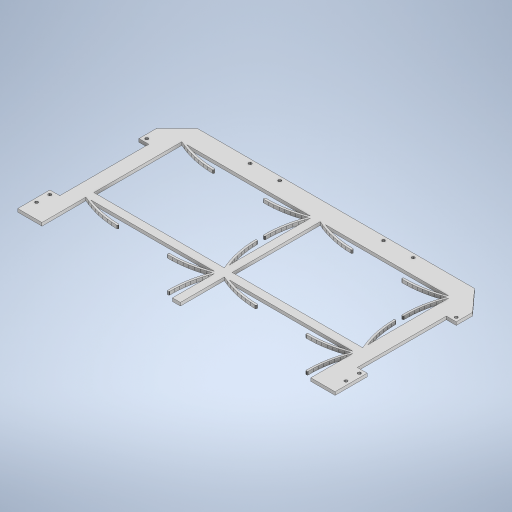
# Autodesk Inventor part: deck_bottom
Saved by Autodesk Inventor 2024.1 (Build 281209000, 209)
## iProperties
Created: 2024-06-24
Part Number: deck_bottom
Material: Generic
Document SubType Name: Modeling
Designer: pab2
Density: 1 g/cm^3
Appearance: Default
Author: pab2
Autodesk Inventor part; units mm, degrees
ref_plane "YZ Plane" through (0, 0, 0) normal (1, 0, 0) x (0, 1, 0)
ref_plane "XZ Plane" through (0, 0, 0) normal (0, 1, 0) x (-1, 0, 0)
ref_plane "XY Plane" through (0, 0, 0) normal (0, 0, 1) x (1, 0, 0)
sketch "Sketch1" plane through (0, 0, 0) normal (0, 1, 0) x (-1, 0, 0)
  line L0 (350.8022, 552.9792) -> (351.4019, 553.085)
  line L1 (351.4019, 553.085) -> (351.8958, 553.4378)
  line L2 (351.8958, 553.4378) -> (352.2133, 553.8964)
  line L3 (352.2133, 553.8964) -> (352.3192, 554.4961)
  line L4 (352.3192, 554.4961) -> (352.2133, 555.0605)
  line L5 (352.2133, 555.0605) -> (351.8958, 555.5544)
  line L6 (351.8958, 555.5544) -> (351.4019, 555.8719)
  line L7 (351.4019, 555.8719) -> (350.8022, 555.9778)
  line L8 (350.8022, 555.9778) -> (350.2378, 555.8719)
  line L9 (350.2378, 555.8719) -> (349.7439, 555.5544)
  line L10 (349.7439, 555.5544) -> (349.4264, 555.0605)
  line L11 (349.4264, 555.0605) -> (349.3206, 554.4961)
  line L12 (349.3206, 554.4961) -> (349.4264, 553.8964)
  line L13 (349.4264, 553.8964) -> (349.7439, 553.4378)
  line L14 (349.7439, 553.4378) -> (350.2378, 553.085)
  line L15 (350.2378, 553.085) -> (350.8022, 552.9792)
  line L16 (320.8161, 552.9792) -> (321.3806, 553.085)
  line L17 (321.3806, 553.085) -> (321.8745, 553.4378)
  line L18 (321.8745, 553.4378) -> (322.1919, 553.8964)
  line L19 (322.1919, 553.8964) -> (322.3331, 554.4961)
  line L20 (322.3331, 554.4961) -> (322.1919, 555.0605)
  line L21 (322.1919, 555.0605) -> (321.8745, 555.5544)
  line L22 (321.8745, 555.5544) -> (321.3806, 555.8719)
  line L23 (321.3806, 555.8719) -> (320.8161, 555.9778)
  line L24 (320.8161, 555.9778) -> (320.2517, 555.8719)
  line L25 (320.2517, 555.8719) -> (319.7578, 555.5544)
  line L26 (319.7578, 555.5544) -> (319.4403, 555.0605)
  line L27 (319.4403, 555.0605) -> (319.3344, 554.4961)
  line L28 (319.3344, 554.4961) -> (319.4403, 553.8964)
  line L29 (319.4403, 553.8964) -> (319.7578, 553.4378)
  line L30 (319.7578, 553.4378) -> (320.2517, 553.085)
  line L31 (320.2517, 553.085) -> (320.8161, 552.9792)
  line L32 (185.8081, 552.9792) -> (186.4078, 553.085)
  line L33 (186.4078, 553.085) -> (186.8664, 553.4378)
  line L34 (186.8664, 553.4378) -> (187.2192, 553.8964)
  line L35 (187.2192, 553.8964) -> (187.325, 554.4961)
  line L36 (187.325, 554.4961) -> (187.2192, 555.0605)
  line L37 (187.2192, 555.0605) -> (186.8664, 555.5544)
  line L38 (186.8664, 555.5544) -> (186.4078, 555.8719)
  line L39 (186.4078, 555.8719) -> (185.8081, 555.9778)
  line L40 (185.8081, 555.9778) -> (185.2436, 555.8719)
  line L41 (185.2436, 555.8719) -> (184.7497, 555.5544)
  line L42 (184.7497, 555.5544) -> (184.4322, 555.0605)
  line L43 (184.4322, 555.0605) -> (184.3264, 554.4961)
  line L44 (184.3264, 554.4961) -> (184.4322, 553.8964)
  line L45 (184.4322, 553.8964) -> (184.7497, 553.4378)
  line L46 (184.7497, 553.4378) -> (185.2436, 553.085)
  line L47 (185.2436, 553.085) -> (185.8081, 552.9792)
  line L48 (224.2961, 577.0033) -> (228.7764, 576.7917)
  line L49 (228.7764, 576.7917) -> (233.2214, 576.4036)
  line L50 (233.2214, 576.4036) -> (237.6664, 575.8391)
  line L51 (237.6664, 575.8391) -> (242.0408, 575.063)
  line L52 (242.0408, 575.063) -> (246.4153, 574.0753)
  line L53 (246.4153, 574.0753) -> (250.7192, 572.9111)
  line L54 (250.7192, 572.9111) -> (254.9878, 571.5353)
  line L55 (254.9878, 571.5353) -> (259.1858, 569.983)
  line L56 (224.3314, 578.9789) -> (223.9433, 578.9083)
  line L57 (223.9433, 578.9083) -> (223.6258, 578.6966)
  line L58 (223.6258, 578.6966) -> (223.4142, 578.3792)
  line L59 (223.4142, 578.3792) -> (223.3083, 577.9911)
  line L60 (223.3083, 577.9911) -> (223.3789, 577.603)
  line L61 (223.3789, 577.603) -> (223.5906, 577.2855)
  line L62 (223.5906, 577.2855) -> (223.9081, 577.0739)
  line L63 (223.9081, 577.0739) -> (224.2961, 577.0033)
  line L64 (264.3011, 569.983) -> (259.5739, 571.9939)
  line L65 (259.5739, 571.9939) -> (254.7056, 573.7577)
  line L66 (254.7056, 573.7577) -> (249.802, 575.2394)
  line L67 (249.802, 575.2394) -> (244.7925, 576.5094)
  line L68 (244.7925, 576.5094) -> (239.7125, 577.5325)
  line L69 (239.7125, 577.5325) -> (234.6325, 578.2733)
  line L70 (234.6325, 578.2733) -> (229.4819, 578.7672)
  line L71 (229.4819, 578.7672) -> (224.3314, 578.9789)
  line L72 (264.3011, 569.983) -> (264.3011, 658.9889)
  line L73 (264.3011, 658.9889) -> (132.327, 658.9889)
  line L74 (141.3228, 619.0191) -> (141.0758, 624.1697)
  line L75 (141.0758, 624.1697) -> (140.5819, 629.285)
  line L76 (140.5819, 629.285) -> (139.8411, 634.4003)
  line L77 (139.8411, 634.4003) -> (138.8533, 639.445)
  line L78 (138.8533, 639.445) -> (137.5833, 644.4544)
  line L79 (137.5833, 644.4544) -> (136.0664, 649.3933)
  line L80 (136.0664, 649.3933) -> (134.3025, 654.2264)
  line L81 (134.3025, 654.2264) -> (132.327, 658.9889)
  line L82 (139.312, 618.9839) -> (139.4178, 618.5958)
  line L83 (139.4178, 618.5958) -> (139.6295, 618.2783)
  line L84 (139.6295, 618.2783) -> (139.9469, 618.0667)
  line L85 (139.9469, 618.0667) -> (140.335, 617.9961)
  line L86 (140.335, 617.9961) -> (140.7231, 618.0667)
  line L87 (140.7231, 618.0667) -> (141.0406, 618.2783)
  line L88 (141.0406, 618.2783) -> (141.2522, 618.6311)
  line L89 (141.2522, 618.6311) -> (141.3228, 619.0191)
  line L90 (132.327, 653.8383) -> (133.8792, 649.6755)
  line L91 (133.8792, 649.6755) -> (135.2197, 645.4069)
  line L92 (135.2197, 645.4069) -> (136.4192, 641.103)
  line L93 (136.4192, 641.103) -> (137.3717, 636.7286)
  line L94 (137.3717, 636.7286) -> (138.1478, 632.3189)
  line L95 (138.1478, 632.3189) -> (138.7475, 627.8739)
  line L96 (138.7475, 627.8739) -> (139.1356, 623.4289)
  line L97 (139.1356, 623.4289) -> (139.312, 618.9839)
  line L98 (132.327, 653.8383) -> (132.327, 572.135)
  line L99 (139.312, 609.988) -> (139.2414, 605.1197)
  line L100 (139.2414, 605.1197) -> (138.9592, 600.2867)
  line L101 (138.9592, 600.2867) -> (138.43, 595.4889)
  line L102 (138.43, 595.4889) -> (137.6539, 590.7264)
  line L103 (137.6539, 590.7264) -> (136.6661, 585.9639)
  line L104 (136.6661, 585.9639) -> (135.4314, 581.3072)
  line L105 (135.4314, 581.3072) -> (133.985, 576.6858)
  line L106 (133.985, 576.6858) -> (132.327, 572.135)
  line L107 (141.3228, 609.988) -> (141.2522, 610.3761)
  line L108 (141.2522, 610.3761) -> (141.0053, 610.6936)
  line L109 (141.0053, 610.6936) -> (140.6878, 610.9053)
  line L110 (140.6878, 610.9053) -> (140.2997, 610.9758)
  line L111 (140.2997, 610.9758) -> (139.9117, 610.9053)
  line L112 (139.9117, 610.9053) -> (139.5942, 610.6936)
  line L113 (139.5942, 610.6936) -> (139.3825, 610.3408)
  line L114 (139.3825, 610.3408) -> (139.312, 609.988)
  line L115 (134.4789, 572.135) -> (136.1017, 576.6858)
  line L116 (136.1017, 576.6858) -> (137.5128, 581.3072)
  line L117 (137.5128, 581.3072) -> (138.7122, 585.9992)
  line L118 (138.7122, 585.9992) -> (139.7, 590.7264)
  line L119 (139.7, 590.7264) -> (140.4408, 595.5242)
  line L120 (140.4408, 595.5242) -> (140.97, 600.3219)
  line L121 (140.97, 600.3219) -> (141.2522, 605.155)
  line L122 (141.2522, 605.155) -> (141.3228, 609.988)
  line L123 (172.332, 578.9789) -> (167.4989, 578.9083)
  line L124 (167.4989, 578.9083) -> (162.6658, 578.6261)
  line L125 (162.6658, 578.6261) -> (157.8681, 578.0969)
  line L126 (157.8681, 578.0969) -> (153.0703, 577.3561)
  line L127 (153.0703, 577.3561) -> (148.3431, 576.4036)
  line L128 (148.3431, 576.4036) -> (143.6511, 575.2042)
  line L129 (143.6511, 575.2042) -> (139.0297, 573.7577)
  line L130 (139.0297, 573.7577) -> (134.4789, 572.135)
  line L131 (172.2967, 576.9681) -> (172.6847, 577.0739)
  line L132 (172.6847, 577.0739) -> (173.0022, 577.2855)
  line L133 (173.0022, 577.2855) -> (173.2492, 577.603)
  line L134 (173.2492, 577.603) -> (173.3197, 577.9911)
  line L135 (173.3197, 577.9911) -> (173.2492, 578.3439)
  line L136 (173.2492, 578.3439) -> (173.0375, 578.6966)
  line L137 (173.0375, 578.6966) -> (172.72, 578.9083)
  line L138 (172.72, 578.9083) -> (172.332, 578.9789)
  line L139 (134.4789, 569.983) -> (138.9944, 571.6411)
  line L140 (138.9944, 571.6411) -> (143.6158, 573.0875)
  line L141 (143.6158, 573.0875) -> (148.3078, 574.3222)
  line L142 (148.3078, 574.3222) -> (153.035, 575.31)
  line L143 (153.035, 575.31) -> (157.8328, 576.0861)
  line L144 (157.8328, 576.0861) -> (162.6306, 576.6153)
  line L145 (162.6306, 576.6153) -> (167.4636, 576.9327)
  line L146 (167.4636, 576.9327) -> (172.2967, 576.9681)
  line L147 (134.4789, 569.983) -> (259.1858, 569.983)
  line L148 (424.815, 694.9722) -> (425.3794, 695.1133)
  line L149 (425.3794, 695.1133) -> (425.8733, 695.4308)
  line L150 (425.8733, 695.4308) -> (426.1908, 695.9247)
  line L151 (426.1908, 695.9247) -> (426.3319, 696.4891)
  line L152 (426.3319, 696.4891) -> (426.1908, 697.0536)
  line L153 (426.1908, 697.0536) -> (425.8733, 697.5475)
  line L154 (425.8733, 697.5475) -> (425.3794, 697.865)
  line L155 (425.3794, 697.865) -> (424.815, 697.9708)
  line L156 (424.815, 697.9708) -> (424.2505, 697.865)
  line L157 (424.2505, 697.865) -> (423.7566, 697.5475)
  line L158 (423.7566, 697.5475) -> (423.4391, 697.0536)
  line L159 (423.4391, 697.0536) -> (423.3333, 696.4891)
  line L160 (423.3333, 696.4891) -> (423.4391, 695.9247)
  line L161 (423.4391, 695.9247) -> (423.7566, 695.4308)
  line L162 (423.7566, 695.4308) -> (424.2505, 695.1133)
  line L163 (424.2505, 695.1133) -> (424.815, 694.9722)
  line L164 (215.8294, 552.9792) -> (216.3939, 553.085)
  line L165 (216.3939, 553.085) -> (216.8878, 553.4378)
  line L166 (216.8878, 553.4378) -> (217.2053, 553.8964)
  line L167 (217.2053, 553.8964) -> (217.3111, 554.4961)
  line L168 (217.3111, 554.4961) -> (217.2053, 555.0605)
  line L169 (217.2053, 555.0605) -> (216.8878, 555.5544)
  line L170 (216.8878, 555.5544) -> (216.3939, 555.8719)
  line L171 (216.3939, 555.8719) -> (215.8294, 555.9778)
  line L172 (215.8294, 555.9778) -> (215.2297, 555.8719)
  line L173 (215.2297, 555.8719) -> (214.7711, 555.5544)
  line L174 (214.7711, 555.5544) -> (214.4183, 555.0605)
  line L175 (214.4183, 555.0605) -> (214.3125, 554.4961)
  line L176 (214.3125, 554.4961) -> (214.4183, 553.8964)
  line L177 (214.4183, 553.8964) -> (214.7711, 553.4378)
  line L178 (214.7711, 553.4378) -> (215.2297, 553.085)
  line L179 (215.2297, 553.085) -> (215.8294, 552.9792)
  line L180 (111.8306, 694.9722) -> (112.395, 695.1133)
  line L181 (112.395, 695.1133) -> (112.8889, 695.4308)
  line L182 (112.8889, 695.4308) -> (113.2064, 695.9247)
  line L183 (113.2064, 695.9247) -> (113.3122, 696.4891)
  line L184 (113.3122, 696.4891) -> (113.2064, 697.0536)
  line L185 (113.2064, 697.0536) -> (112.8889, 697.5475)
  line L186 (112.8889, 697.5475) -> (112.395, 697.865)
  line L187 (112.395, 697.865) -> (111.8306, 697.9708)
  line L188 (111.8306, 697.9708) -> (111.2309, 697.865)
  line L189 (111.2309, 697.865) -> (110.7722, 697.5475)
  line L190 (110.7722, 697.5475) -> (110.4194, 697.0536)
  line L191 (110.4194, 697.0536) -> (110.3136, 696.4891)
  line L192 (110.3136, 696.4891) -> (110.4194, 695.9247)
  line L193 (110.4194, 695.9247) -> (110.7722, 695.4308)
  line L194 (110.7722, 695.4308) -> (111.2309, 695.1133)
  line L195 (111.2309, 695.1133) -> (111.8306, 694.9722)
  line L196 (364.3136, 577.0033) -> (368.7586, 576.7917)
  line L197 (368.7586, 576.7917) -> (373.2036, 576.4036)
  line L198 (373.2036, 576.4036) -> (377.6486, 575.8391)
  line L199 (377.6486, 575.8391) -> (382.0583, 575.063)
  line L200 (382.0583, 575.063) -> (386.4328, 574.0753)
  line L201 (386.4328, 574.0753) -> (390.7367, 572.9111)
  line L202 (390.7367, 572.9111) -> (395.0053, 571.5353)
  line L203 (395.0053, 571.5353) -> (399.2033, 569.983)
  line L204 (364.3489, 578.9789) -> (363.9608, 578.9083)
  line L205 (363.9608, 578.9083) -> (363.608, 578.6966)
  line L206 (363.608, 578.6966) -> (363.3964, 578.3792)
  line L207 (363.3964, 578.3792) -> (363.3258, 577.9911)
  line L208 (363.3258, 577.9911) -> (363.3964, 577.603)
  line L209 (363.3964, 577.603) -> (363.608, 577.2855)
  line L210 (363.608, 577.2855) -> (363.9255, 577.0739)
  line L211 (363.9255, 577.0739) -> (364.3136, 577.0033)
  line L212 (404.3186, 569.983) -> (399.5561, 571.9939)
  line L213 (399.5561, 571.9939) -> (394.7231, 573.7577)
  line L214 (394.7231, 573.7577) -> (389.7842, 575.2394)
  line L215 (389.7842, 575.2394) -> (384.7747, 576.5094)
  line L216 (384.7747, 576.5094) -> (379.73, 577.5325)
  line L217 (379.73, 577.5325) -> (374.6147, 578.2733)
  line L218 (374.6147, 578.2733) -> (369.4995, 578.7672)
  line L219 (369.4995, 578.7672) -> (364.3489, 578.9789)
  line L220 (404.3186, 569.983) -> (404.3186, 658.9889)
  line L221 (404.3186, 658.9889) -> (272.3092, 658.9889)
  line L222 (281.305, 619.0191) -> (281.0933, 624.1697)
  line L223 (281.0933, 624.1697) -> (280.5995, 629.285)
  line L224 (280.5995, 629.285) -> (279.8586, 634.4003)
  line L225 (279.8586, 634.4003) -> (278.8356, 639.445)
  line L226 (278.8356, 639.445) -> (277.6008, 644.4544)
  line L227 (277.6008, 644.4544) -> (276.0839, 649.3933)
  line L228 (276.0839, 649.3933) -> (274.32, 654.2264)
  line L229 (274.32, 654.2264) -> (272.3092, 658.9889)
  line L230 (279.3294, 618.9839) -> (279.4, 618.5958)
  line L231 (279.4, 618.5958) -> (279.6117, 618.2783)
  line L232 (279.6117, 618.2783) -> (279.9644, 618.0667)
  line L233 (279.9644, 618.0667) -> (280.3525, 617.9961)
  line L234 (280.3525, 617.9961) -> (280.7053, 618.0667)
  line L235 (280.7053, 618.0667) -> (281.0228, 618.2783)
  line L236 (281.0228, 618.2783) -> (281.2344, 618.6311)
  line L237 (281.2344, 618.6311) -> (281.305, 619.0191)
  line L238 (272.3092, 653.8383) -> (273.8614, 649.6755)
  line L239 (273.8614, 649.6755) -> (275.2372, 645.4069)
  line L240 (275.2372, 645.4069) -> (276.4014, 641.103)
  line L241 (276.4014, 641.103) -> (277.3892, 636.7286)
  line L242 (277.3892, 636.7286) -> (278.1653, 632.3189)
  line L243 (278.1653, 632.3189) -> (278.765, 627.8739)
  line L244 (278.765, 627.8739) -> (279.1178, 623.4289)
  line L245 (279.1178, 623.4289) -> (279.3294, 618.9839)
  line L246 (272.3092, 653.8383) -> (272.3092, 572.135)
  line L247 (279.3294, 609.988) -> (279.2589, 605.1197)
  line L248 (279.2589, 605.1197) -> (278.9414, 600.2867)
  line L249 (278.9414, 600.2867) -> (278.4122, 595.4889)
  line L250 (278.4122, 595.4889) -> (277.6714, 590.7264)
  line L251 (277.6714, 590.7264) -> (276.6483, 585.9639)
  line L252 (276.6483, 585.9639) -> (275.4489, 581.3072)
  line L253 (275.4489, 581.3072) -> (274.0025, 576.6858)
  line L254 (274.0025, 576.6858) -> (272.3092, 572.135)
  line L255 (281.305, 609.988) -> (281.2344, 610.3761)
  line L256 (281.2344, 610.3761) -> (281.0228, 610.6936)
  line L257 (281.0228, 610.6936) -> (280.7053, 610.9053)
  line L258 (280.7053, 610.9053) -> (280.3172, 610.9758)
  line L259 (280.3172, 610.9758) -> (279.9292, 610.9053)
  line L260 (279.9292, 610.9053) -> (279.6117, 610.6936)
  line L261 (279.6117, 610.6936) -> (279.4, 610.3408)
  line L262 (279.4, 610.3408) -> (279.3294, 609.988)
  line L263 (274.4611, 572.135) -> (276.1192, 576.6858)
  line L264 (276.1192, 576.6858) -> (277.5303, 581.3072)
  line L265 (277.5303, 581.3072) -> (278.7297, 585.9992)
  line L266 (278.7297, 585.9992) -> (279.6822, 590.7264)
  line L267 (279.6822, 590.7264) -> (280.4583, 595.5242)
  line L268 (280.4583, 595.5242) -> (280.9522, 600.3219)
  line L269 (280.9522, 600.3219) -> (281.2697, 605.155)
  line L270 (281.2697, 605.155) -> (281.305, 609.988)
  line L271 (312.3142, 578.9789) -> (307.4811, 578.9083)
  line L272 (307.4811, 578.9083) -> (302.6481, 578.6261)
  line L273 (302.6481, 578.6261) -> (297.8503, 578.0969)
  line L274 (297.8503, 578.0969) -> (293.0878, 577.3561)
  line L275 (293.0878, 577.3561) -> (288.3253, 576.4036)
  line L276 (288.3253, 576.4036) -> (283.6333, 575.2042)
  line L277 (283.6333, 575.2042) -> (279.012, 573.7577)
  line L278 (279.012, 573.7577) -> (274.4611, 572.135)
  line L279 (312.3142, 576.9681) -> (312.7022, 577.0739)
  line L280 (312.7022, 577.0739) -> (313.0197, 577.2855)
  line L281 (313.0197, 577.2855) -> (313.2314, 577.603)
  line L282 (313.2314, 577.603) -> (313.3019, 577.9911)
  line L283 (313.3019, 577.9911) -> (313.2314, 578.3439)
  line L284 (313.2314, 578.3439) -> (313.0197, 578.6966)
  line L285 (313.0197, 578.6966) -> (312.7022, 578.9083)
  line L286 (312.7022, 578.9083) -> (312.3142, 578.9789)
  line L287 (274.4611, 569.983) -> (279.012, 571.6411)
  line L288 (279.012, 571.6411) -> (283.6333, 573.0875)
  line L289 (283.6333, 573.0875) -> (288.3253, 574.3222)
  line L290 (288.3253, 574.3222) -> (293.0525, 575.31)
  line L291 (293.0525, 575.31) -> (297.815, 576.0861)
  line L292 (297.815, 576.0861) -> (302.6481, 576.6153)
  line L293 (302.6481, 576.6153) -> (307.4811, 576.9327)
  line L294 (307.4811, 576.9327) -> (312.3142, 576.9681)
  line L295 (274.4611, 569.983) -> (399.2033, 569.983)
  line L296 (111.8306, 583.4239) -> (112.395, 583.565)
  line L297 (112.395, 583.565) -> (112.8889, 583.8825)
  line L298 (112.8889, 583.8825) -> (113.2064, 584.3764)
  line L299 (113.2064, 584.3764) -> (113.3122, 584.9408)
  line L300 (113.3122, 584.9408) -> (113.2064, 585.5053)
  line L301 (113.2064, 585.5053) -> (112.8889, 585.9992)
  line L302 (112.8889, 585.9992) -> (112.395, 586.3167)
  line L303 (112.395, 586.3167) -> (111.8306, 586.4225)
  line L304 (111.8306, 586.4225) -> (111.2309, 586.3167)
  line L305 (111.2309, 586.3167) -> (110.7722, 585.9992)
  line L306 (110.7722, 585.9992) -> (110.4194, 585.5053)
  line L307 (110.4194, 585.5053) -> (110.3136, 584.9408)
  line L308 (110.3136, 584.9408) -> (110.4194, 584.3764)
  line L309 (110.4194, 584.3764) -> (110.7722, 583.8825)
  line L310 (110.7722, 583.8825) -> (111.2309, 583.565)
  line L311 (111.2309, 583.565) -> (111.8306, 583.4239)
  line L312 (407.8111, 550.4744) -> (428.8014, 571.5)
  line L313 (127.8114, 550.4744) -> (407.8111, 550.4744)
  line L314 (107.8089, 572.4525) -> (127.8114, 550.4744)
  line L315 (107.8089, 588.9272) -> (107.8089, 572.4525)
  line L316 (107.8089, 588.9272) -> (117.8278, 588.9272)
  line L317 (117.8278, 588.9272) -> (117.8278, 678.9561)
  line L318 (117.8278, 678.9561) -> (107.8089, 678.9561)
  line L319 (132.327, 711.4822) -> (107.8089, 711.4822)
  line L320 (132.327, 669.1489) -> (132.327, 711.4822)
  line L321 (139.312, 706.9667) -> (139.2414, 702.1336)
  line L322 (139.2414, 702.1336) -> (138.9592, 697.3005)
  line L323 (138.9592, 697.3005) -> (138.43, 692.5028)
  line L324 (138.43, 692.5028) -> (137.6539, 687.705)
  line L325 (137.6539, 687.705) -> (136.6661, 682.9778)
  line L326 (136.6661, 682.9778) -> (135.4314, 678.2858)
  line L327 (135.4314, 678.2858) -> (133.985, 673.6644)
  line L328 (133.985, 673.6644) -> (132.327, 669.1489)
  line L329 (141.3228, 707.0019) -> (141.2522, 707.39)
  line L330 (141.2522, 707.39) -> (141.0053, 707.7075)
  line L331 (141.0053, 707.7075) -> (140.6878, 707.9191)
  line L332 (140.6878, 707.9191) -> (140.2997, 707.9897)
  line L333 (140.2997, 707.9897) -> (139.9117, 707.9191)
  line L334 (139.9117, 707.9191) -> (139.5942, 707.6722)
  line L335 (139.5942, 707.6722) -> (139.3825, 707.3547)
  line L336 (139.3825, 707.3547) -> (139.312, 706.9667)
  line L337 (134.4789, 669.1489) -> (136.1017, 673.6997)
  line L338 (136.1017, 673.6997) -> (137.5128, 678.3211)
  line L339 (137.5128, 678.3211) -> (138.7122, 683.013)
  line L340 (138.7122, 683.013) -> (139.7, 687.7403)
  line L341 (139.7, 687.7403) -> (140.4408, 692.5028)
  line L342 (140.4408, 692.5028) -> (140.97, 697.3358)
  line L343 (140.97, 697.3358) -> (141.2522, 702.1689)
  line L344 (141.2522, 702.1689) -> (141.3228, 707.0019)
  line L345 (172.332, 675.9928) -> (167.4989, 675.9222)
  line L346 (167.4989, 675.9222) -> (162.6658, 675.64)
  line L347 (162.6658, 675.64) -> (157.8681, 675.1108)
  line L348 (157.8681, 675.1108) -> (153.0703, 674.37)
  line L349 (153.0703, 674.37) -> (148.3431, 673.3822)
  line L350 (148.3431, 673.3822) -> (143.6511, 672.1827)
  line L351 (143.6511, 672.1827) -> (139.0297, 670.7716)
  line L352 (139.0297, 670.7716) -> (134.4789, 669.1489)
  line L353 (172.2967, 673.9819) -> (172.6847, 674.0525)
  line L354 (172.6847, 674.0525) -> (173.0022, 674.2641)
  line L355 (173.0022, 674.2641) -> (173.2492, 674.5816)
  line L356 (173.2492, 674.5816) -> (173.3197, 674.9697)
  line L357 (173.3197, 674.9697) -> (173.2492, 675.3577)
  line L358 (173.2492, 675.3577) -> (173.0375, 675.6753)
  line L359 (173.0375, 675.6753) -> (172.72, 675.9222)
  line L360 (172.72, 675.9222) -> (172.332, 675.9928)
  line L361 (134.4789, 666.9969) -> (138.9944, 668.655)
  line L362 (138.9944, 668.655) -> (143.6158, 670.1014)
  line L363 (143.6158, 670.1014) -> (148.3078, 671.3361)
  line L364 (148.3078, 671.3361) -> (153.035, 672.3239)
  line L365 (153.035, 672.3239) -> (157.8328, 673.1)
  line L366 (157.8328, 673.1) -> (162.6306, 673.6292)
  line L367 (162.6306, 673.6292) -> (167.4636, 673.9114)
  line L368 (167.4636, 673.9114) -> (172.2967, 673.9819)
  line L369 (259.1858, 666.9969) -> (134.4789, 666.9969)
  line L370 (224.2961, 673.9819) -> (228.7764, 673.8056)
  line L371 (228.7764, 673.8056) -> (233.2214, 673.4175)
  line L372 (233.2214, 673.4175) -> (237.6664, 672.8178)
  line L373 (237.6664, 672.8178) -> (242.0408, 672.0417)
  line L374 (242.0408, 672.0417) -> (246.4153, 671.0891)
  line L375 (246.4153, 671.0891) -> (250.7192, 669.8897)
  line L376 (250.7192, 669.8897) -> (254.9878, 668.5492)
  line L377 (254.9878, 668.5492) -> (259.1858, 666.9969)
  line L378 (224.3314, 675.9928) -> (223.9433, 675.9222)
  line L379 (223.9433, 675.9222) -> (223.6258, 675.7105)
  line L380 (223.6258, 675.7105) -> (223.4142, 675.3931)
  line L381 (223.4142, 675.3931) -> (223.3083, 675.005)
  line L382 (223.3083, 675.005) -> (223.3789, 674.6169)
  line L383 (223.3789, 674.6169) -> (223.5906, 674.2994)
  line L384 (223.5906, 674.2994) -> (223.9081, 674.0525)
  line L385 (223.9081, 674.0525) -> (224.2961, 673.9819)
  line L386 (264.3011, 666.9969) -> (259.5739, 668.9725)
  line L387 (259.5739, 668.9725) -> (254.7056, 670.7364)
  line L388 (254.7056, 670.7364) -> (249.802, 672.2533)
  line L389 (249.802, 672.2533) -> (244.7925, 673.5233)
  line L390 (244.7925, 673.5233) -> (239.7125, 674.5111)
  line L391 (239.7125, 674.5111) -> (234.6325, 675.2519)
  line L392 (234.6325, 675.2519) -> (229.4819, 675.7458)
  line L393 (229.4819, 675.7458) -> (224.3314, 675.9928)
  line L394 (264.3011, 711.4822) -> (264.3011, 666.9969)
  line L395 (272.3092, 711.4822) -> (264.3011, 711.4822)
  line L396 (272.3092, 669.1489) -> (272.3092, 711.4822)
  line L397 (279.3294, 706.9667) -> (279.2589, 702.1336)
  line L398 (279.2589, 702.1336) -> (278.9414, 697.3005)
  line L399 (278.9414, 697.3005) -> (278.4122, 692.5028)
  line L400 (278.4122, 692.5028) -> (277.6714, 687.705)
  line L401 (277.6714, 687.705) -> (276.6483, 682.9778)
  line L402 (276.6483, 682.9778) -> (275.4489, 678.2858)
  line L403 (275.4489, 678.2858) -> (274.0025, 673.6644)
  line L404 (274.0025, 673.6644) -> (272.3092, 669.1489)
  line L405 (281.305, 707.0019) -> (281.2344, 707.39)
  line L406 (281.2344, 707.39) -> (281.0228, 707.7075)
  line L407 (281.0228, 707.7075) -> (280.7053, 707.9191)
  line L408 (280.7053, 707.9191) -> (280.3172, 707.9897)
  line L409 (280.3172, 707.9897) -> (279.9292, 707.9191)
  line L410 (279.9292, 707.9191) -> (279.6117, 707.6722)
  line L411 (279.6117, 707.6722) -> (279.4, 707.3547)
  line L412 (279.4, 707.3547) -> (279.3294, 706.9667)
  line L413 (274.4611, 669.1489) -> (276.1192, 673.6997)
  line L414 (276.1192, 673.6997) -> (277.5303, 678.3211)
  line L415 (277.5303, 678.3211) -> (278.7297, 683.013)
  line L416 (278.7297, 683.013) -> (279.6822, 687.7403)
  line L417 (279.6822, 687.7403) -> (280.4583, 692.5028)
  line L418 (280.4583, 692.5028) -> (280.9522, 697.3358)
  line L419 (280.9522, 697.3358) -> (281.2697, 702.1689)
  line L420 (281.2697, 702.1689) -> (281.305, 707.0019)
  line L421 (312.3142, 675.9928) -> (307.4811, 675.9222)
  line L422 (307.4811, 675.9222) -> (302.6481, 675.64)
  line L423 (302.6481, 675.64) -> (297.8503, 675.1108)
  line L424 (297.8503, 675.1108) -> (293.0878, 674.37)
  line L425 (293.0878, 674.37) -> (288.3253, 673.3822)
  line L426 (288.3253, 673.3822) -> (283.6333, 672.1827)
  line L427 (283.6333, 672.1827) -> (279.012, 670.7716)
  line L428 (279.012, 670.7716) -> (274.4611, 669.1489)
  line L429 (312.3142, 673.9819) -> (312.7022, 674.0525)
  line L430 (312.7022, 674.0525) -> (313.0197, 674.2641)
  line L431 (313.0197, 674.2641) -> (313.2314, 674.5816)
  line L432 (313.2314, 674.5816) -> (313.3019, 674.9697)
  line L433 (313.3019, 674.9697) -> (313.2314, 675.3577)
  line L434 (313.2314, 675.3577) -> (313.0197, 675.6753)
  line L435 (313.0197, 675.6753) -> (312.7022, 675.9222)
  line L436 (312.7022, 675.9222) -> (312.3142, 675.9928)
  line L437 (274.4611, 666.9969) -> (279.012, 668.655)
  line L438 (279.012, 668.655) -> (283.6333, 670.1014)
  line L439 (283.6333, 670.1014) -> (288.3253, 671.3361)
  line L440 (288.3253, 671.3361) -> (293.0525, 672.3239)
  line L441 (293.0525, 672.3239) -> (297.815, 673.1)
  line L442 (297.815, 673.1) -> (302.6481, 673.6292)
  line L443 (302.6481, 673.6292) -> (307.4811, 673.9114)
  line L444 (307.4811, 673.9114) -> (312.3142, 673.9819)
  line L445 (399.2033, 666.9969) -> (274.4611, 666.9969)
  line L446 (364.3136, 673.9819) -> (368.7586, 673.8056)
  line L447 (368.7586, 673.8056) -> (373.2036, 673.4175)
  line L448 (373.2036, 673.4175) -> (377.6486, 672.8178)
  line L449 (377.6486, 672.8178) -> (382.0583, 672.0417)
  line L450 (382.0583, 672.0417) -> (386.4328, 671.0891)
  line L451 (386.4328, 671.0891) -> (390.7367, 669.8897)
  line L452 (390.7367, 669.8897) -> (395.0053, 668.5492)
  line L453 (395.0053, 668.5492) -> (399.2033, 666.9969)
  line L454 (364.3489, 675.9928) -> (363.9608, 675.9222)
  line L455 (363.9608, 675.9222) -> (363.608, 675.7105)
  line L456 (363.608, 675.7105) -> (363.3964, 675.3931)
  line L457 (363.3964, 675.3931) -> (363.3258, 675.005)
  line L458 (363.3258, 675.005) -> (363.3964, 674.6169)
  line L459 (363.3964, 674.6169) -> (363.608, 674.2994)
  line L460 (363.608, 674.2994) -> (363.9255, 674.0525)
  line L461 (363.9255, 674.0525) -> (364.3136, 673.9819)
  line L462 (404.3186, 666.9969) -> (399.5561, 668.9725)
  line L463 (399.5561, 668.9725) -> (394.7231, 670.7364)
  line L464 (394.7231, 670.7364) -> (389.7842, 672.2533)
  line L465 (389.7842, 672.2533) -> (384.7747, 673.5233)
  line L466 (384.7747, 673.5233) -> (379.73, 674.5111)
  line L467 (379.73, 674.5111) -> (374.6147, 675.2519)
  line L468 (374.6147, 675.2519) -> (369.4995, 675.7458)
  line L469 (369.4995, 675.7458) -> (364.3489, 675.9928)
  line L470 (404.3186, 711.4822) -> (404.3186, 666.9969)
  line L471 (428.8014, 711.4822) -> (404.3186, 711.4822)
  line L472 (428.8014, 678.9561) -> (428.8014, 711.4822)
  line L473 (428.8014, 678.9561) -> (418.8178, 678.9561)
  line L474 (418.8178, 678.9561) -> (418.8178, 588.9272)
  line L475 (418.8178, 588.9272) -> (428.8014, 588.9272)
  line L476 (111.8306, 681.4255) -> (112.395, 681.5667)
  line L477 (112.395, 681.5667) -> (112.8889, 681.8841)
  line L478 (112.8889, 681.8841) -> (113.2064, 682.378)
  line L479 (113.2064, 682.378) -> (113.3122, 682.9425)
  line L480 (113.3122, 682.9425) -> (113.2064, 683.5069)
  line L481 (113.2064, 683.5069) -> (112.8889, 684.0008)
  line L482 (112.8889, 684.0008) -> (112.395, 684.3183)
  line L483 (112.395, 684.3183) -> (111.8306, 684.4242)
  line L484 (111.8306, 684.4242) -> (111.2309, 684.3183)
  line L485 (111.2309, 684.3183) -> (110.7722, 684.0008)
  line L486 (110.7722, 684.0008) -> (110.4194, 683.5069)
  line L487 (110.4194, 683.5069) -> (110.3136, 682.9425)
  line L488 (110.3136, 682.9425) -> (110.4194, 682.378)
  line L489 (110.4194, 682.378) -> (110.7722, 681.8841)
  line L490 (110.7722, 681.8841) -> (111.2309, 681.5667)
  line L491 (111.2309, 681.5667) -> (111.8306, 681.4255)
  line L492 (424.815, 681.4255) -> (425.3794, 681.5667)
  line L493 (425.3794, 681.5667) -> (425.8733, 681.8841)
  line L494 (425.8733, 681.8841) -> (426.1908, 682.378)
  line L495 (426.1908, 682.378) -> (426.3319, 682.9425)
  line L496 (426.3319, 682.9425) -> (426.1908, 683.5069)
  line L497 (426.1908, 683.5069) -> (425.8733, 684.0008)
  line L498 (425.8733, 684.0008) -> (425.3794, 684.3183)
  line L499 (425.3794, 684.3183) -> (424.815, 684.4242)
  line L500 (424.815, 684.4242) -> (424.2505, 684.3183)
  line L501 (424.2505, 684.3183) -> (423.7566, 684.0008)
  line L502 (423.7566, 684.0008) -> (423.4391, 683.5069)
  line L503 (423.4391, 683.5069) -> (423.3333, 682.9425)
  line L504 (423.3333, 682.9425) -> (423.4391, 682.378)
  line L505 (423.4391, 682.378) -> (423.7566, 681.8841)
  line L506 (423.7566, 681.8841) -> (424.2505, 681.5667)
  line L507 (424.2505, 681.5667) -> (424.815, 681.4255)
  line L508 (424.815, 583.4239) -> (425.3794, 583.565)
  line L509 (425.3794, 583.565) -> (425.8733, 583.8825)
  line L510 (425.8733, 583.8825) -> (426.1908, 584.3764)
  line L511 (426.1908, 584.3764) -> (426.3319, 584.9408)
  line L512 (426.3319, 584.9408) -> (426.1908, 585.5053)
  line L513 (426.1908, 585.5053) -> (425.8733, 585.9992)
  line L514 (425.8733, 585.9992) -> (425.3794, 586.3167)
  line L515 (425.3794, 586.3167) -> (424.815, 586.4225)
  line L516 (424.815, 586.4225) -> (424.2505, 586.3167)
  line L517 (424.2505, 586.3167) -> (423.7566, 585.9992)
  line L518 (423.7566, 585.9992) -> (423.4391, 585.5053)
  line L519 (423.4391, 585.5053) -> (423.3333, 584.9408)
  line L520 (423.3333, 584.9408) -> (423.4391, 584.3764)
  line L521 (423.4391, 584.3764) -> (423.7566, 583.8825)
  line L522 (423.7566, 583.8825) -> (424.2505, 583.565)
  line L523 (424.2505, 583.565) -> (424.815, 583.4239)
  line L524 (428.8014, 571.5) -> (428.8014, 588.9272)
  line L525 (107.8089, 711.4822) -> (107.8089, 678.9561)
  point P0 (0, 0)
  constraints: 1052 end point
extrude "Extrusion1" add sketch "Sketch1" along normal blind 3.175
body "Solid1"
